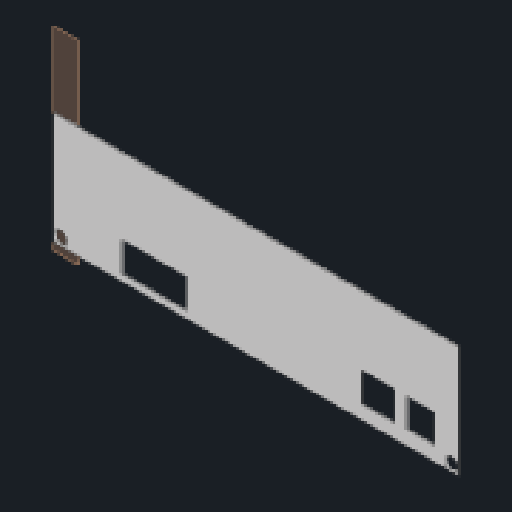
# Autodesk Inventor part: ceil_front
Saved by Autodesk Inventor 2023 (Build 270158000, 158)
## iProperties
Created: 2024-04-28
Part Number: ceil_front
Material: ABS Plastic
Document SubType Name: Modeling
Designer: szymo
Density: 1.06 g/cm^3
Appearance: Smooth - White
Mass: 4.84401 g
Surface Area: 157.179 cm^2
Volume: 4.56982 cm^3
Author: szymo
Autodesk Inventor part; units mm, degrees
ref_plane "YZ Plane" through (0, 0, 0) normal (1, 0, 0) x (0, 1, 0)
ref_plane "XZ Plane" through (0, 0, 0) normal (0, 1, 0) x (-1, 0, 0)
ref_plane "XY Plane" through (0, 0, 0) normal (0, 0, 1) x (1, 0, 0)
ref_plane "Work Plane1" through (0, 0, 0) normal (0, 0, 1) x (1, 0, 0)
sketch "Sketch1" plane through (0, 0, 0) normal (0, 0, 1) x (1, 0, 0)
  line L0 (84.5, 12.4325) -> (84.5, -11.5675) projected
  line L1 (84.5, -11.5675) -> (72.5, -11.5675) projected
  line L2 (72.5, -11.5675) -> (72.5, 4.5875) projected
  circle A0 centre (69.5, 4.5875) radius 3 projected
  line L3 (72.5, 4.5875) -> (72.5, 12.4325) projected
  line L4 (72.5, 12.4325) -> (84.5, 12.4325) projected
  arc A1 (105.5, 4.2836) -> (105.5, 4.8914) centre (108.4846, 4.5875) ccw projected
  line L5 (105.5, 4.2836) -> (105.5, -11.5675) projected
  line L6 (105.5, -11.5675) -> (93.5, -11.5675) projected
  line L7 (93.5, -11.5675) -> (93.5, 12.4325) projected
  line L8 (93.5, 12.4325) -> (105.5, 12.4325) projected
  line L9 (105.5, 12.4325) -> (105.5, 4.8914) projected
  circle A2 centre (108.4462, 27.5) radius 3 projected
  circle A3 centre (69.5, 27.5) radius 3 projected
  circle A4 centre (89, 0.9661) radius 3 projected
  circle A5 centre (89, 29.5) radius 3 projected
  arc A6 (175, 0) -> (178, -3) centre (175, -3) ccw projected
  line L10 (175, 0) -> (115.0397, 0) projected
  line L11 (65.5, 33.8) -> (65.5, 0) projected
  line L12 (65.5, 0) -> (65.1397, 0) projected
  arc A7 (0, -3) -> (3, 0) centre (3, -3) ccw projected
  line L13 (0, -3) -> (0, -25.75) projected
  arc A8 (3, -28.75) -> (0, -25.75) centre (3, -25.75) ccw projected
  line L14 (3, -28.75) -> (62.9603, -28.75) projected
  arc A9 (178, -25.75) -> (175, -28.75) centre (175, -25.75) ccw projected
  line L15 (178, -25.75) -> (178, -3) projected
  circle A10 centre (3, -25.75) radius 2.3 projected
  circle A11 centre (3, -3) radius 2.3 projected
  circle A12 centre (3, -74.8889) radius 2.3 projected
  line L16 (0, 0) -> (6, 0) projected
  line L17 (0, -77.8889) -> (0, 0) projected
  line L18 (0, -77.8889) -> (6, -77.8889) projected
  line L19 (6, -71.8889) -> (6, -77.8889) projected
  line L20 (6, -71.8889) -> (1.6, -71.8889) projected
  line L21 (1.6, -71.8889) -> (1.6, -56.7889) projected
  line L22 (1.6, -56.7889) -> (3, -56.7889) projected
  line L23 (3, -28.75) -> (3, -56.7889) projected
  line L24 (3, -28.75) -> (6, -28.75) projected
  line L25 (6, -28.75) -> (6, -22.75) projected
  line L26 (6, -22.75) -> (3, -22.75) projected
  line L27 (3, -6) -> (3, -22.75) projected
  line L28 (3, -6) -> (6, -6) projected
  line L29 (6, -6) -> (6, 0) projected
  circle A13 centre (175, -3) radius 2.3 projected
  circle A14 centre (175, -25.75) radius 2.3 projected
  line L30 (175, -28.75) -> (175, -71.8889) projected
  line L31 (175, -6) -> (175, -22.75) projected
  line L32 (175, -71.8889) -> (172, -71.8889) projected
  line L33 (172, -71.8889) -> (172, -77.8889) projected
  line L34 (178, -77.8889) -> (172, -77.8889) projected
  line L35 (178, -77.8889) -> (178, 0) projected
  line L36 (178, 0) -> (172, 0) projected
  line L37 (172, 0) -> (172, -6) projected
  line L38 (172, -6) -> (175, -6) projected
  line L39 (175, -22.75) -> (172, -22.75) projected
  line L40 (172, -22.75) -> (172, -28.75) projected
  line L41 (172, -28.75) -> (175, -28.75) projected
  circle A15 centre (175, -74.8889) radius 2.3 projected
  line L42 (156.2, -70.4889) -> (156.2, -59.9889) projected
  line L43 (166.7, -59.9889) -> (156.2, -59.9889) projected
  line L44 (166.7, -59.9889) -> (166.7, -70.4889) projected
  line L45 (156.2, -70.4889) -> (166.7, -70.4889) projected
  line L46 (149, -59.8889) -> (149, -70.8889) projected
  line L47 (149, -70.8889) -> (136.35, -70.8889) projected
  line L48 (136.35, -70.8889) -> (136.35, -59.8889) projected
  line L49 (136.35, -59.8889) -> (149, -59.8889) projected
  line L50 (135, -53.8889) -> (135, -71.8889) projected
  line L51 (135, -71.8889) -> (175, -71.8889) projected
  line L52 (175, -71.8889) -> (175, -53.8889) projected
  line L53 (175, -53.8889) -> (135, -53.8889) projected
  circle A16 centre (137.85, -56.7389) radius 1.5 projected
  circle A17 centre (172.15, -56.7389) radius 1.5 projected
  line L54 (31.25, -62.8889) -> (31.25, -73.8889) projected
  line L55 (31.25, -73.8889) -> (57.25, -73.8889) projected
  line L56 (57.25, -73.8889) -> (57.25, -62.8889) projected
  line L57 (57.25, -62.8889) -> (31.25, -62.8889) projected
  line L58 (3, -56.7889) -> (23.3, -56.7889) projected
  line L59 (23.3, -56.7889) -> (23.3, -59.8889) projected
  line L60 (23.3, -59.8889) -> (23.3, -65.1889) projected
  line L61 (3, -71.8889) -> (23.3, -71.8889) projected
  line L62 (23.3, -61.8889) -> (23.3, -74.8889) projected
  line L63 (30.25, -61.8889) -> (30.25, -74.8889)
  line L64 (30.25, -74.8889) -> (58.25, -74.8889)
  line L65 (58.25, -74.8889) -> (58.25, -61.8889)
  line L66 (58.25, -61.8889) -> (30.25, -61.8889)
  line L67 (150, -58.8889) -> (150, -71.8889)
  line L68 (150, -71.8889) -> (135.35, -71.8889)
  line L69 (135.35, -71.8889) -> (135.35, -58.8889)
  line L70 (135.35, -58.8889) -> (150, -58.8889)
  line L71 (155.2, -58.9889) -> (155.2, -71.4889)
  line L72 (155.2, -71.4889) -> (167.7, -71.4889)
  line L73 (167.7, -71.4889) -> (167.7, -58.9889)
  line L74 (167.7, -58.9889) -> (155.2, -58.9889)
  line L75 (0, -28.75) -> (178, -28.75)
  line L76 (178, -28.75) -> (178, -77.8889)
  line L77 (178, -77.8889) -> (0, -77.8889)
  line L78 (0, -77.8889) -> (0, -28.75)
  line L79 (131.125, -21.1625) -> (131.125, -7.525) projected
  arc A18 (134.125, -4.525) -> (131.125, -7.525) centre (134.125, -7.525) ccw projected
  line L80 (134.125, -4.525) -> (155.95, -4.525) projected
  arc A19 (158.95, -7.525) -> (155.95, -4.525) centre (155.95, -7.525) ccw projected
  line L81 (158.95, -7.525) -> (158.95, -21.1625) projected
  arc A20 (155.95, -24.1625) -> (158.95, -21.1625) centre (155.95, -21.1625) ccw projected
  line L82 (155.95, -24.1625) -> (134.125, -24.1625) projected
  arc A21 (131.125, -21.1625) -> (134.125, -24.1625) centre (134.125, -21.1625) ccw projected
  line L83 (46.875, -7.5875) -> (46.875, -21.225) projected
  arc A22 (43.875, -24.225) -> (46.875, -21.225) centre (43.875, -21.225) ccw projected
  line L84 (43.875, -24.225) -> (22.05, -24.225) projected
  arc A23 (19.05, -21.225) -> (22.05, -24.225) centre (22.05, -21.225) ccw projected
  line L85 (19.05, -21.225) -> (19.05, -7.5875) projected
  arc A24 (22.05, -4.5875) -> (19.05, -7.5875) centre (22.05, -7.5875) ccw projected
  line L86 (22.05, -4.5875) -> (43.875, -4.5875) projected
  arc A25 (46.875, -7.5875) -> (43.875, -4.5875) centre (43.875, -7.5875) ccw projected
  line L87 (112.5, 0) -> (112.5, 33.8) projected
  line L88 (112.5, 33.8) -> (65.5, 33.8) projected
  arc A26 (115.0397, -28.75) -> (112.8603, -28.75) centre (113.95, -26.5) ccw projected
  line L89 (115.0397, -28.75) -> (175, -28.75) projected
  arc A27 (112.8603, 0) -> (115.0397, 0) centre (113.95, -2.25) ccw projected
  line L90 (112.8603, 0) -> (112.5, 0) projected
  arc A28 (62.9603, 0) -> (65.1397, 0) centre (64.05, -2.25) ccw projected
  line L91 (62.9603, 0) -> (3, 0) projected
  arc A29 (65.1397, -28.75) -> (62.9603, -28.75) centre (64.05, -26.5) ccw projected
  line L92 (65.1397, -28.75) -> (112.8603, -28.75) projected
  point P0 (168.4, -53.8889)
  point P1 (135.35, -71.8889)
  point P2 (6, -25.75)
  point P3 (3, -28.75)
  dimension "d0" = 1
  dimension "d1" = 1
  dimension "d2" = 1
  constraints: 32 end point, 2 parallel, 1 horizontal, 1 horizontal alignment, 1 perpendicular, 1 point on line, 9 other
  measures "d0" distance between parallel lines of L57 L66
  measures "d1" distance between parallel lines of L49 L70
  measures "d2" distance between parallel lines of L43 L74
extrude "Extrusion1" add sketch "Sketch1" along normal blind 0.6 contours L35 L34 L33 L32 L30 L75 | L30 L53 L50 L51 L33 L77 L19 L61 L62 L60 L59 L58 L23 L14 L75 L41 | L30 L32 L51 L67 L70 L69 L50 L53 | L18 L17 L75 L23 L22 L21 L20 L19 | L20 L21 L22 L58 L59 L60 L62 L61 | A12 | A15 | A16 | A17
sketch "Sketch2" plane through (0, 0, 0.6) normal (0, 0, 1) x (1, 0, 0)
  circle A0 centre (3, -25.75) radius 2.3 projected
  circle A1 centre (3, -3) radius 2.3 projected
  circle A2 centre (3, -74.8889) radius 2.3 projected
  line L0 (0, 0) -> (6, 0) projected
  line L1 (0, -77.8889) -> (0, 0) projected
  line L2 (0, -77.8889) -> (6, -77.8889) projected
  line L3 (6, -71.8889) -> (6, -77.8889) projected
  line L4 (6, -71.8889) -> (1.6, -71.8889) projected
  line L5 (1.6, -71.8889) -> (1.6, -56.7889) projected
  line L6 (1.6, -56.7889) -> (3, -56.7889) projected
  line L7 (3, -28.75) -> (3, -56.7889) projected
  line L8 (3, -28.75) -> (6, -28.75) projected
  line L9 (6, -28.75) -> (6, -22.75) projected
  line L10 (6, -22.75) -> (3, -22.75) projected
  line L11 (3, -6) -> (3, -22.75) projected
  line L12 (3, -6) -> (6, -6) projected
  line L13 (6, -6) -> (6, 0) projected
  circle A3 centre (175, -3) radius 2.3 projected
  circle A4 centre (175, -25.75) radius 2.3 projected
  line L14 (175, -28.75) -> (175, -71.8889) projected
  line L15 (175, -6) -> (175, -22.75) projected
  line L16 (175, -71.8889) -> (172, -71.8889) projected
  line L17 (172, -71.8889) -> (172, -77.8889) projected
  line L18 (178, -77.8889) -> (172, -77.8889) projected
  line L19 (178, -77.8889) -> (178, 0) projected
  line L20 (178, 0) -> (172, 0) projected
  line L21 (172, 0) -> (172, -6) projected
  line L22 (172, -6) -> (175, -6) projected
  line L23 (175, -22.75) -> (172, -22.75) projected
  line L24 (172, -22.75) -> (172, -28.75) projected
  line L25 (172, -28.75) -> (175, -28.75) projected
  circle A5 centre (175, -74.8889) radius 2.3 projected
  constraints: 2 coincident
hole "Hole1" at (3, -74.8889, 0.6) at (175, -74.8889, 0.6) direction (0, 0, -1) diameter 3.6 end through all countersink diameter 6 countersink angle 90 clearance for "Countersunk Flat Head Screw ISO 2009/7046" size "M3" standard "ISO"
body "Solid1"
